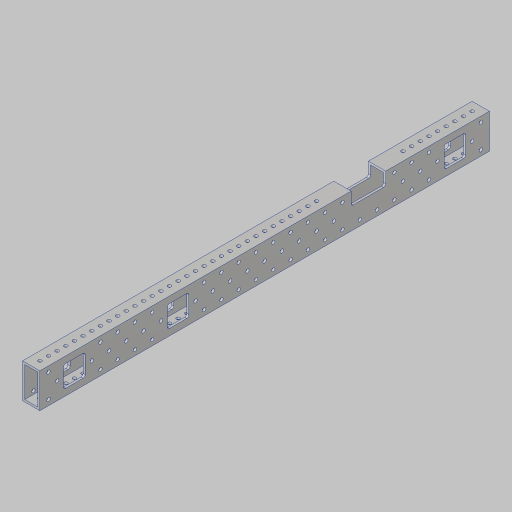
# Autodesk Inventor part: DB1-002
Saved by Autodesk Inventor 2023.5 (Build 275446000, 446)
## iProperties
RuleStatus: InUse
Created: 2025-01-09
Part Number: DB1-002
Material: Aluminum 6061
Document SubType Name: Modeling
Designer: mavericks
Mass: 679.915 g
Surface Area: 1725.81 cm^2
Volume: 251.82 cm^3
Density: 2.7 g/cm^3
Appearance: Aluminum - Flat
AfterDocNew0: SHOW
AfterDocOpen0: SHOW
Author: mavericks
Autodesk Inventor part; units mm, degrees
ref_plane "YZ Plane" through (0, 0, 0) normal (1, 0, 0) x (0, 1, 0)
ref_plane "XZ Plane" through (0, 0, 0) normal (0, 1, 0) x (-1, 0, 0)
ref_plane "XY Plane" through (0, 0, 0) normal (0, 0, 1) x (1, 0, 0)
sketch "Sketch1" plane through (0, 0, 0) normal (0, 0, 1) x (1, 0, 0)
  line L0 (-12.7, -25.4) -> (12.7, -25.4)
  line L1 (12.7, -25.4) -> (12.7, 25.4)
  line L2 (12.7, 25.4) -> (-12.7, 25.4)
  line L3 (-12.7, 25.4) -> (-12.7, -25.4)
  line L4 (-12.7, -25.4) -> (12.7, 25.4) construction
  line L5 (12.7, -25.4) -> (-12.7, 25.4) construction
  line L6 (-9.525, 22.225) -> (9.525, 22.225)
  line L7 (9.525, 22.225) -> (9.525, -22.225)
  line L8 (9.525, -22.225) -> (-9.525, -22.225)
  line L9 (-9.525, -22.225) -> (-9.525, 22.225)
  point P0 (0, 0)
  dimension "width" = 25.4
  dimension "height" = 50.8
  dimension "thickness" = 3.175
  constraints: 20 end point, 4 parallel, 2 midpoint, 2 perpendicular, 1 horizontal, 3 other
  measures "width" distance of L2.end L1.end
  measures "height" distance of L1.end L0.end
  measures "thickness" distance between parallel lines of L2 L6
extrude "Extrusion1" add sketch "Sketch1" along normal mid plane 660.4
sketch "Sketch2" plane through (-12.7, 25.4, 330.2) normal (0, 1, 0) x (1, 0, 0)
  line L0 (12.7, 342.9) -> (12.7, 317.5) construction
  line L1 (0, 660.4) -> (0, 0) construction
  point P0 (12.7, 330.2)
  point P1 (12.7, 330.2)
  point P2 (12.7, 304.8)
  point P3 (12.7, 292.1)
  point P4 (12.7, 279.4)
  point P5 (12.7, 266.7)
  point P6 (12.7, 254)
  point P7 (12.7, 241.3)
  point P8 (12.7, 228.6)
  point P9 (12.7, 215.9)
  point P10 (12.7, 203.2)
  point P11 (12.7, 190.5)
  point P12 (12.7, 177.8)
  point P13 (12.7, 165.1)
  point P14 (12.7, 152.4)
  point P15 (12.7, 139.7)
  point P16 (12.7, 127)
  point P17 (12.7, 114.3)
  point P18 (12.7, 101.6)
  point P19 (12.7, 88.9)
  point P20 (12.7, 76.2)
  point P21 (12.7, 63.5)
  point P22 (12.7, 50.8)
  point P23 (12.7, 38.1)
  point P24 (12.7, 25.4)
  point P25 (12.7, 355.6)
  point P26 (12.7, 368.3)
  point P27 (12.7, 381)
  point P28 (12.7, 393.7)
  point P29 (12.7, 406.4)
  point P30 (12.7, 419.1)
  point P31 (12.7, 431.8)
  point P32 (12.7, 444.5)
  point P33 (12.7, 457.2)
  point P34 (12.7, 469.9)
  point P35 (12.7, 482.6)
  point P36 (12.7, 495.3)
  point P37 (12.7, 508)
  point P38 (12.7, 520.7)
  point P39 (12.7, 533.4)
  point P40 (12.7, 546.1)
  point P41 (12.7, 558.8)
  point P42 (12.7, 571.5)
  point P43 (12.7, 584.2)
  point P44 (12.7, 596.9)
  point P45 (12.7, 609.6)
  point P46 (12.7, 622.3)
  point P47 (12.7, 635)
  point P48 (12.7, 330.2)
  point P49 (12.7, 647.7)
  point P50 (12.7, 12.7)
  dimension "d6" = 25.4
  dimension "d9" = 12.7
  dimension "d16" = 12.7
  constraints: 3 vertical, 2 coincident, 2 end point, 2 vertical alignment, 1 midpoint, 48 other
  measures "d6" distance of L0.start L0.end
  measures "d9" distance of L0.end point (12.7, 304.8)
  measures "d16" distance of L0.start point (12.7, 355.6)
hole "Hole1" at (0, 25.4, 12.7) at (0, 25.4, -12.7) at (0, 25.4, 25.4) at (0, 25.4, 38.1) at (0, 25.4, 50.8) at (0, 25.4, 63.5) at (0, 25.4, 76.2) at (0, 25.4, 88.9) at (0, 25.4, 101.6) at (0, 25.4, 114.3) at (0, 25.4, 127) at (0, 25.4, 139.7) at (0, 25.4, 152.4) at (0, 25.4, 165.1) at (0, 25.4, 177.8) at (0, 25.4, 190.5) at (0, 25.4, 203.2) at (0, 25.4, 215.9) at (0, 25.4, 228.6) at (0, 25.4, 241.3) at (0, 25.4, 254) at (0, 25.4, 266.7) at (0, 25.4, 279.4) at (0, 25.4, 292.1) at (0, 25.4, 304.8) at (0, 25.4, -25.4) at (0, 25.4, -38.1) at (0, 25.4, -50.8) at (0, 25.4, -63.5) at (0, 25.4, -76.2) at (0, 25.4, -88.9) at (0, 25.4, -215.9) at (0, 25.4, -228.6) at (0, 25.4, -241.3) at (0, 25.4, -254) at (0, 25.4, -266.7) at (0, 25.4, -279.4) at (0, 25.4, -292.1) at (0, 25.4, -304.8) at (0, 25.4, 0) at (0, 25.4, 317.5) at (0, 25.4, -317.5) direction (0, -1, 0) diameter 5.1054 end through all clearance for "Flat Head Machine Screw (82)" size "#10" standard "Ansi Unified Screw Threads"
sketch "Sketch3" plane through (12.7, -25.4, 330.2) normal (1, 0, 0) x (0, 0, -1)
  line L0 (317.5, 42.8625) -> (317.5, 7.9375) construction
  circle A0 centre (317.5, 42.8625) radius 4.7625 construction
  line L1 (0, 47.625) -> (660.4, 47.625) construction
  circle A1 centre (317.5, 7.9375) radius 4.7625 construction
  line L2 (0, 3.175) -> (660.4, 3.175) construction
  line L3 (317.5, 42.8625) -> (342.9, 42.8625) construction
  point P0 (330.2, 25.4)
  point P1 (330.2, 25.4)
  point P2 (342.9, 7.9375)
  point P3 (292.1, 42.8625)
  point P4 (304.8, 25.4)
  point P5 (292.1, 7.9375)
  point P6 (266.7, 42.8625)
  point P7 (279.4, 25.4)
  point P8 (266.7, 7.9375)
  point P9 (241.3, 42.8625)
  point P10 (254, 25.4)
  point P11 (241.3, 7.9375)
  point P12 (215.9, 42.8625)
  point P13 (228.6, 25.4)
  point P14 (215.9, 7.9375)
  point P15 (190.5, 42.8625)
  point P16 (203.2, 25.4)
  point P17 (190.5, 7.9375)
  point P18 (165.1, 42.8625)
  point P19 (177.8, 25.4)
  point P20 (165.1, 7.9375)
  point P21 (139.7, 42.8625)
  point P22 (152.4, 25.4)
  point P23 (139.7, 7.9375)
  point P24 (114.3, 42.8625)
  point P25 (127, 25.4)
  point P26 (114.3, 7.9375)
  point P27 (88.9, 42.8625)
  point P28 (101.6, 25.4)
  point P29 (88.9, 7.9375)
  point P30 (63.5, 42.8625)
  point P31 (76.2, 25.4)
  point P32 (63.5, 7.9375)
  point P33 (38.1, 42.8625)
  point P34 (50.8, 25.4)
  point P35 (38.1, 7.9375)
  point P36 (12.7, 42.8625)
  point P37 (25.4, 25.4)
  point P38 (12.7, 7.9375)
  point P39 (355.6, 25.4)
  point P40 (355.6, 25.4)
  point P41 (368.3, 42.8625)
  point P42 (368.3, 7.9375)
  point P43 (381, 25.4)
  point P44 (381, 25.4)
  point P45 (393.7, 42.8625)
  point P46 (393.7, 7.9375)
  point P47 (406.4, 25.4)
  point P48 (406.4, 25.4)
  point P49 (419.1, 42.8625)
  point P50 (419.1, 7.9375)
  point P51 (431.8, 25.4)
  point P52 (431.8, 25.4)
  point P53 (444.5, 42.8625)
  point P54 (444.5, 7.9375)
  point P55 (457.2, 25.4)
  point P56 (457.2, 25.4)
  point P57 (469.9, 42.8625)
  point P58 (469.9, 7.9375)
  point P59 (482.6, 25.4)
  point P60 (482.6, 25.4)
  point P61 (495.3, 42.8625)
  point P62 (495.3, 7.9375)
  point P63 (508, 25.4)
  point P64 (508, 25.4)
  point P65 (520.7, 42.8625)
  point P66 (520.7, 7.9375)
  point P67 (533.4, 25.4)
  point P68 (533.4, 25.4)
  point P69 (546.1, 42.8625)
  point P70 (546.1, 7.9375)
  point P71 (558.8, 25.4)
  point P72 (558.8, 25.4)
  point P73 (571.5, 42.8625)
  point P74 (571.5, 7.9375)
  point P75 (584.2, 25.4)
  point P76 (584.2, 25.4)
  point P77 (596.9, 42.8625)
  point P78 (596.9, 7.9375)
  point P79 (609.6, 25.4)
  point P80 (609.6, 25.4)
  point P81 (622.3, 42.8625)
  point P82 (622.3, 7.9375)
  point P83 (635, 25.4)
  point P84 (635, 25.4)
  point P85 (647.7, 42.8625)
  point P86 (647.7, 7.9375)
  dimension "d28" = 12.7
  dimension "d29" = 9.525
  dimension "d30" = 9.525
  dimension "d31" = 25.4
  dimension "d34" = 25.4
  dimension "d41" = 25.4
  constraints: 17 coincident, 4 end point, 3 horizontal, 2 centre point, 2 horizontal alignment, 2 tangent, 2 vertical alignment, 1 vertical, 84 other
  measures "d28" horizontal distance of point (330.2, 25.4) L0.start
  measures "d29" diameter of A0
  measures "d30" diameter of A1
  measures "d31" distance of L3.end L3.start
  measures "d34" distance of L0.start point (292.1, 42.863)
  measures "d41" distance of point (330.2, 25.4) point (355.6, 25.4)
hole "Hole2" at (12.7, 0, 0) at (12.7, 17.4625, 12.7) at (12.7, 17.4625, -12.7) at (12.7, -17.4625, -12.7) at (12.7, -17.4625, 12.7) at (12.7, 17.4625, 38.1) at (12.7, 0, 25.4) at (12.7, -17.4625, 38.1) at (12.7, 17.4625, 63.5) at (12.7, 0, 50.8) at (12.7, -17.4625, 63.5) at (12.7, 17.4625, 88.9) at (12.7, 0, 76.2) at (12.7, -17.4625, 88.9) at (12.7, 0, 101.6) at (12.7, 0, 127) at (12.7, 17.4625, 165.1) at (12.7, 0, 152.4) at (12.7, -17.4625, 165.1) at (12.7, 17.4625, 190.5) at (12.7, 0, 177.8) at (12.7, -17.4625, 190.5) at (12.7, 17.4625, 215.9) at (12.7, 0, 203.2) at (12.7, -17.4625, 215.9) at (12.7, 17.4625, 241.3) at (12.7, 0, 228.6) at (12.7, -17.4625, 241.3) at (12.7, 0, 254) at (12.7, 0, 279.4) at (12.7, 17.4625, 317.5) at (12.7, 0, 304.8) at (12.7, -17.4625, 317.5) at (12.7, 0, -25.4) at (12.7, 17.4625, -38.1) at (12.7, -17.4625, -38.1) at (12.7, 0, -50.8) at (12.7, 17.4625, -63.5) at (12.7, -17.4625, -63.5) at (12.7, 0, -76.2) at (12.7, 17.4625, -88.9) at (12.7, -17.4625, -88.9) at (12.7, 0, -101.6) at (12.7, -17.4625, -165.1) at (12.7, -17.4625, -190.5) at (12.7, 0, -203.2) at (12.7, -17.4625, -215.9) at (12.7, 0, -228.6) at (12.7, 17.4625, -241.3) at (12.7, -17.4625, -241.3) direction (-1, 0, 0) diameter 5.1054 end through all and at (12.7, 0, -254) (12.7, 0, -279.4) (12.7, 0, -304.8) (12.7, 17.4625, -317.5) (12.7, -17.4625, -317.5) (12.7, -17.4625, -139.7) (12.7, -17.4625, -114.3) (12.7, 17.4625, -215.9) (12.7, 17.4625, -190.5) (12.7, 17.4625, -114.3) clearance for "Flat Head Machine Screw (82)" size "#10" standard "Ansi Unified Screw Threads"
sketch "Sketch5" plane through (12.7, -25.4, 330.2) normal (1, 0, 0) x (0, 0, -1)
  line L0 (34.925, 41.275) -> (66.675, 41.275)
  line L1 (66.675, 41.275) -> (66.675, 9.525)
  line L2 (66.675, 9.525) -> (34.925, 9.525)
  line L3 (34.925, 9.525) -> (34.925, 41.275)
  circle A0 centre (50.8, 25.4) radius 2.5527 projected
  line L4 (34.925, 41.275) -> (66.675, 9.525) construction
  line L5 (66.675, 41.275) -> (34.925, 9.525) construction
  line L6 (593.725, 41.275) -> (625.475, 41.275)
  line L7 (625.475, 41.275) -> (625.475, 9.525)
  line L8 (625.475, 9.525) -> (593.725, 9.525)
  line L9 (593.725, 9.525) -> (593.725, 41.275)
  circle A1 centre (609.6, 25.4) radius 2.5527
  line L10 (593.725, 41.275) -> (625.475, 9.525) construction
  line L11 (625.475, 41.275) -> (593.725, 9.525) construction
  circle A2 centre (584.2, 25.4) radius 2.5527 projected
  circle A3 centre (203.2, 25.4) radius 2.5527 projected
  line L12 (187.325, 41.275) -> (219.075, 41.275)
  line L13 (219.075, 41.275) -> (219.075, 9.525)
  line L14 (219.075, 9.525) -> (187.325, 9.525)
  line L15 (187.325, 9.525) -> (187.325, 41.275)
  circle A4 centre (203.2, 25.4) radius 2.5527 projected
  line L16 (187.325, 41.275) -> (219.075, 9.525) construction
  line L17 (219.075, 41.275) -> (187.325, 9.525) construction
  circle A5 centre (609.6, 25.4) radius 2.5527 projected
  point P0 (330.2, 25.4)
  dimension "d59" = 31.75
  dimension "d60" = 31.75
  constraints: 36 end point, 6 midpoint, 6 parallel, 4 equal length, 3 horizontal, 3 perpendicular, 1 centre point, 1 coincident
  measures "d59" distance of L0.start L0.end
  measures "d60" distance of L0.end L1.end
extrude "Extrusion3" cut sketch "Sketch5" against normal blind 25.4 contours L0 L1 L2 L3 | A0 | L6 L7 L8 L9 | L12 L13 L14 L15
fillet "Fillet1" radius 3.175 24 edges at (11.1125, -15.875, 263.525) (11.1125, 15.875, 263.525) (11.1125, 15.875, 295.275) (11.1125, -15.875, 295.275) (-11.1125, -15.875, 295.275) (-11.1125, 15.875, 263.525) (-11.1125, 15.875, 295.275) (-11.1125, -15.875, 263.525) (11.1125, -15.875, -295.275) (-11.1125, -15.875, -295.275) (11.1125, 15.875, -295.275) (11.1125, 15.875, -263.525) (11.1125, -15.875, -263.525) (-11.1125, 15.875, -295.275) (-11.1125, 15.875, -263.525) (-11.1125, -15.875, -263.525) (11.1125, -15.875, 111.125) (11.1125, 15.875, 111.125) (11.1125, 15.875, 142.875) (11.1125, -15.875, 142.875) (-11.1125, -15.875, 142.875) (-11.1125, 15.875, 142.875) (-11.1125, 15.875, 111.125) (-11.1125, -15.875, 111.125)
sketch "Sketch6" plane through (-12.7, -25.4, 330.2) normal (-1, 0, 0) x (0, 0, 1)
  arc A0 (-622.3, 41.275) -> (-625.475, 38.1) centre (-622.3, 38.1) ccw projected
  line L0 (-625.475, 38.1) -> (-625.475, 12.7) projected
  arc A1 (-625.475, 12.7) -> (-622.3, 9.525) centre (-622.3, 12.7) ccw projected
  line L1 (-622.3, 9.525) -> (-596.9, 9.525) projected
  arc A2 (-596.9, 9.525) -> (-593.725, 12.7) centre (-596.9, 12.7) ccw projected
  line L2 (-593.725, 12.7) -> (-593.725, 38.1) projected
  arc A3 (-593.725, 38.1) -> (-596.9, 41.275) centre (-596.9, 38.1) ccw projected
  line L3 (-596.9, 41.275) -> (-622.3, 41.275) projected
  arc A4 (-34.925, 38.1) -> (-38.1, 41.275) centre (-38.1, 38.1) ccw projected
  line L4 (-38.1, 41.275) -> (-63.5, 41.275) projected
  arc A5 (-63.5, 41.275) -> (-66.675, 38.1) centre (-63.5, 38.1) ccw projected
  line L5 (-66.675, 38.1) -> (-66.675, 12.7) projected
  arc A6 (-66.675, 12.7) -> (-63.5, 9.525) centre (-63.5, 12.7) ccw projected
  line L6 (-63.5, 9.525) -> (-38.1, 9.525) projected
  arc A7 (-38.1, 9.525) -> (-34.925, 12.7) centre (-38.1, 12.7) ccw projected
  line L7 (-34.925, 12.7) -> (-34.925, 38.1) projected
  circle A8 centre (-469.9, 7.9375) radius 2.5527 projected
  circle A9 centre (-647.7, 42.8625) radius 2.5527 projected
  circle A10 centre (-571.5, 7.9375) radius 2.5527 projected
  circle A11 centre (-558.8, 25.4) radius 2.5527 projected
  circle A12 centre (-520.7, 7.9375) radius 2.5527 projected
  circle A13 centre (-419.1, 7.9375) radius 2.5527 projected
  circle A14 centre (-406.4, 25.4) radius 2.5527 projected
  circle A15 centre (-393.7, 42.8625) radius 2.5527 projected
  circle A16 centre (-368.3, 7.9375) radius 2.5527 projected
  circle A17 centre (-355.6, 25.4) radius 2.5527 projected
  circle A18 centre (-25.4, 25.4) radius 2.5527 projected
  circle A19 centre (-88.9, 7.9375) radius 2.5527 projected
  circle A20 centre (-88.9, 42.8625) radius 2.5527 projected
  circle A21 centre (-127, 25.4) radius 2.5527 projected
  circle A22 centre (-139.7, 7.9375) radius 2.5527 projected
  circle A23 centre (-139.7, 42.8625) radius 2.5527 projected
  circle A24 centre (-177.8, 25.4) radius 2.5527 projected
  circle A25 centre (-241.3, 7.9375) radius 2.5527 projected
  circle A26 centre (-241.3, 42.8625) radius 2.5527 projected
  circle A27 centre (-279.4, 25.4) radius 2.5527 projected
  circle A28 centre (-292.1, 7.9375) radius 2.5527 projected
  circle A29 centre (-292.1, 42.8625) radius 2.5527 projected
  circle A30 centre (-342.9, 7.9375) radius 2.5527 projected
  circle A31 centre (-317.5, 42.8625) radius 2.5527 projected
  circle A32 centre (-330.2, 25.4) radius 2.5527 projected
  circle A33 centre (-342.9, 42.8625) radius 2.5527 projected
  circle A34 centre (-317.5, 7.9375) radius 2.5527 projected
  circle A35 centre (-304.8, 25.4) radius 2.5527 projected
  circle A36 centre (-266.7, 42.8625) radius 2.5527 projected
  circle A37 centre (-266.7, 7.9375) radius 2.5527 projected
  circle A38 centre (-254, 25.4) radius 2.5527 projected
  circle A39 centre (-228.6, 25.4) radius 2.5527 projected
  circle A40 centre (-165.1, 42.8625) radius 2.5527 projected
  circle A41 centre (-165.1, 7.9375) radius 2.5527 projected
  circle A42 centre (-152.4, 25.4) radius 2.5527 projected
  circle A43 centre (-114.3, 42.8625) radius 2.5527 projected
  circle A44 centre (-114.3, 7.9375) radius 2.5527 projected
  circle A45 centre (-101.6, 25.4) radius 2.5527 projected
  circle A46 centre (-76.2, 25.4) radius 2.5527 projected
  circle A47 centre (-12.7, 42.8625) radius 2.5527 projected
  circle A48 centre (-12.7, 7.9375) radius 2.5527 projected
  circle A49 centre (-368.3, 42.8625) radius 2.5527 projected
  circle A50 centre (-381, 25.4) radius 2.5527 projected
  circle A51 centre (-393.7, 7.9375) radius 2.5527 projected
  circle A52 centre (-419.1, 42.8625) radius 2.5527 projected
  circle A53 centre (-431.8, 25.4) radius 2.5527 projected
  circle A54 centre (-495.3, 7.9375) radius 2.5527 projected
  circle A55 centre (-533.4, 25.4) radius 2.5527 projected
  circle A56 centre (-546.1, 7.9375) radius 2.5527 projected
  circle A57 centre (-571.5, 42.8625) radius 2.5527 projected
  circle A58 centre (-584.2, 25.4) radius 2.5527 projected
  circle A59 centre (-635, 25.4) radius 2.5527 projected
  circle A60 centre (-647.7, 7.9375) radius 2.5527 projected
  circle A61 centre (-444.5, 7.9375) radius 2.5527 projected
  line L8 (-660.4, 0) -> (-660.4, 50.8) projected
  line L9 (-660.4, 50.8) -> (0, 50.8) projected
  line L10 (0, 50.8) -> (0, 0) projected
  line L11 (0, 0) -> (-660.4, 0) projected
  line L12 (-660.4, 50.8) -> (0, 50.8) projected
  line L13 (-508, 50.8) -> (-508, 31.75)
  line L14 (-508, 31.75) -> (-457.2, 31.75)
  line L15 (-457.2, 31.75) -> (-457.2, 50.8)
  line L16 (-508, 50.8) -> (-457.2, 50.8)
  circle A62 centre (-546.1, 42.8625) radius 2.5527 projected
  circle A63 centre (-520.7, 42.8625) radius 2.5527 projected
  circle A64 centre (-444.5, 42.8625) radius 2.5527 projected
  arc A65 (-219.075, 12.7) -> (-215.9, 9.525) centre (-215.9, 12.7) ccw projected
  line L17 (-215.9, 9.525) -> (-190.5, 9.525) projected
  arc A66 (-190.5, 9.525) -> (-187.325, 12.7) centre (-190.5, 12.7) ccw projected
  line L18 (-187.325, 12.7) -> (-187.325, 38.1) projected
  arc A67 (-187.325, 38.1) -> (-190.5, 41.275) centre (-190.5, 38.1) ccw projected
  line L19 (-190.5, 41.275) -> (-215.9, 41.275) projected
  arc A68 (-215.9, 41.275) -> (-219.075, 38.1) centre (-215.9, 38.1) ccw projected
  line L20 (-219.075, 38.1) -> (-219.075, 12.7) projected
  dimension "d64" = 152.4
  dimension "d66" = 19.05
  dimension "d67" = 50.8
  constraints: 8 end point, 2 parallel, 2 point on line, 1 vertical
  measures "d64" distance of L8.end L13.start
  measures "d66" distance between parallel lines of L9 L14
  measures "d67" distance of L13.end L14.end
extrude "Extrusion4" cut sketch "Sketch6" against normal blind 25.4 contours L9 L15 L14 L13
fillet "Fillet2" radius 3.175 4 edges at (-11.1125, 6.35, -177.8) (11.1125, 6.35, -177.8) (11.1125, 6.35, -127) (-11.1125, 6.35, -127)
body "Solid1"
